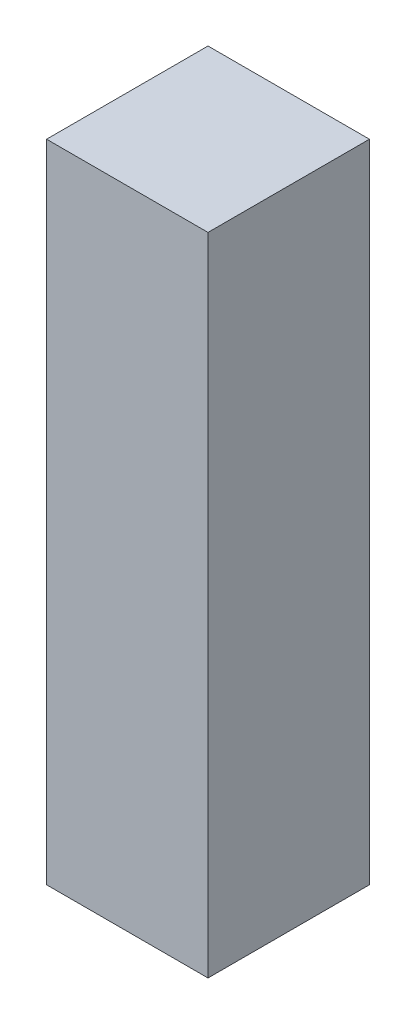
# Autodesk Inventor part: HatchArmGripperFingers
Saved by Autodesk Inventor 2018 (Build 220112000, 112)
## iProperties
Created: 2019-01-08
Part Number: HatchArmGripperFingers
Material: Generic
Document SubType Name: Modeling
Designer: Gabriel
Density: 1 g/cm^3
Appearance: Default
Author: Gabriel
Autodesk Inventor part; units mm, degrees
ref_plane "YZ Plane" through (0, 0, 0) normal (1, 0, 0) x (0, 1, 0)
ref_plane "XZ Plane" through (0, 0, 0) normal (0, 1, 0) x (-1, 0, 0)
ref_plane "XY Plane" through (0, 0, 0) normal (0, 0, 1) x (1, 0, 0)
sketch "Sketch1" plane through (0, 0, 0) normal (0, 0, 1) x (1, 0, 0)
  line L0 (-25.7101, 10.2815) -> (-0.3101, 10.2815)
  line L1 (-0.3101, 10.2815) -> (-0.3101, -91.3185)
  line L2 (-0.3101, -91.3185) -> (-25.7101, -91.3185)
  line L3 (-25.7101, -91.3185) -> (-25.7101, 10.2815)
  point P0 (0, 0)
  dimension "d0" = 25.4
  dimension "d1" = 101.6
  constraints: 8 end point, 2 parallel, 1 horizontal, 1 perpendicular
  measures "d0" distance of L1.end L2.end
  measures "d1" distance of L0.end L1.end
extrude "Extrusion1" add sketch "Sketch1" along normal blind 25.4
body "Solid1"
